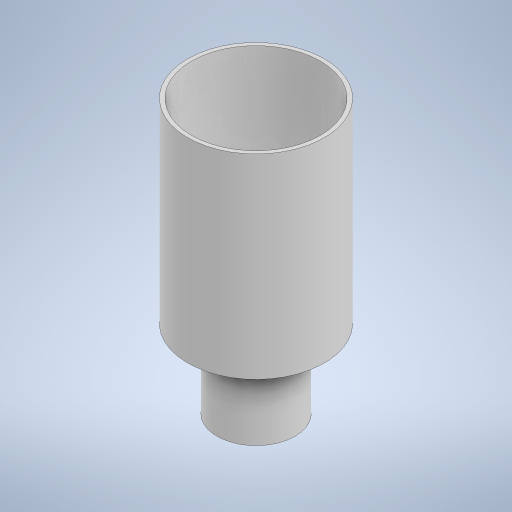
# Autodesk Inventor part: new seed container
Saved by Autodesk Inventor 2023 (Build 270158000, 158)
## iProperties
Created: 2022-06-26
Part Number: new seed container
Material: Generic
Document SubType Name: Modeling
Designer: Shivan
Density: 1 g/cm^3
Appearance: Default
Author: Shivan
Autodesk Inventor part; units mm, degrees
ref_plane "YZ Plane" through (0, 0, 0) normal (1, 0, 0) x (0, 1, 0)
ref_plane "XZ Plane" through (0, 0, 0) normal (0, 1, 0) x (-1, 0, 0)
ref_plane "XY Plane" through (0, 0, 0) normal (0, 0, 1) x (1, 0, 0)
sketch "Sketch1" plane through (0, 0, 0) normal (0, 1, 0) x (-1, 0, 0)
  circle A0 centre (0, 0) radius 17.5
  circle A1 centre (0, 0) radius 10
  dimension "d0" = 35
  dimension "d1" = 20
  constraints: 2 centre point, 2 coincident
  measures "d0" diameter of A0
  measures "d1" diameter of A1
extrude "Extrusion1" add sketch "Sketch1" along normal blind 50 contours A0 | A1
extrude "Extrusion2" add sketch "Sketch1" against normal blind 20 contours A1
shell "Shell1" thickness 1 removed faces 1 at (-4.3663, 50, -1.0762)
sketch "Sketch2" plane through (0, -20, 0) normal (0, -1, 0) x (1, 0, 0)
  point P0 (0, 0)
  point P1 (0, 0)
  constraints: 1 coincident
hole "Hole1" at (0, -20, 0) direction (0, 1, 0) diameter 19.5 depth 50
body "Solid1"
